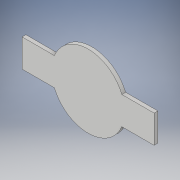
# Autodesk Inventor part: Emblem
Saved by Autodesk Inventor 2019.3 (Build 233278000, 278)
## iProperties
Created: 2020-09-20
Part Number: Emblem
Material: Generisch
Document SubType Name: Modeling
Designer: Nicolas Frick
Density: 1 g/cm^3
Appearance: Vorgabe
Author: Nicolas Frick
Autodesk Inventor part; units mm, degrees
ref_plane "YZ Plane" through (0, 0, 0) normal (1, 0, 0) x (0, 1, 0)
ref_plane "XZ Plane" through (0, 0, 0) normal (0, 1, 0) x (-1, 0, 0)
ref_plane "XY Plane" through (0, 0, 0) normal (0, 0, 1) x (1, 0, 0)
sketch "Skizze1" plane through (0, 0, 0) normal (0, 0, 1) x (1, 0, 0)
  line L0 (-50, 9) -> (-50, -9) construction
  line L1 (50, 9) -> (50, -9) construction
  line L2 (-50, -9) -> (-50, 9)
  line L3 (-50, 9) -> (-25.1982, 9)
  line L4 (25.1982, 9) -> (50, 9)
  line L5 (50, -9) -> (25.1982, -9)
  line L6 (-25.1982, -9) -> (-50, -9)
  line L7 (50, 9) -> (29.5255, 5.3146) construction
  arc A0 (25.1982, 9) -> (-25.1982, 9) centre (0, 0) ccw
  arc A1 (-25.1982, -9) -> (25.1982, -9) centre (0, 0) ccw
  line L8 (50, -12.5) -> (50, -9) construction
  line L9 (50, 9) -> (50, 12.5) construction
  line L10 (50, 9) -> (50, -9)
  point P0 (0, 0)
  dimension "d13" = 100
  dimension "d14" = 18
  constraints: 22 end point, 7 parallel, 4 point on circle, 2 centre point, 2 horizontal, 2 perpendicular, 1 coincident, 1 collinear
  measures "d13" distance of L0.end L1.end
  measures "d14" distance of L1.start L1.end
extrude "Extrusion1" add sketch "Skizze1" along normal blind 3
sketch "Skizze3" plane through (0, 0, 0) normal (0, 0, -1) x (-1, 0, 0)
  line L0 (50, -12.5) -> (50, 12.5) construction
  line L1 (50, 12.5) -> (27.2718, 12.5) construction
  arc A0 (27.2718, 12.5) -> (-27.2718, 12.5) centre (0, 0) ccw construction
  line L2 (-27.2718, 12.5) -> (-50, 12.5) construction
  line L3 (-50, 12.5) -> (-50, -12.5) construction
  line L4 (-50, -12.5) -> (-27.2718, -12.5) construction
  arc A1 (-27.2718, -12.5) -> (27.2718, -12.5) centre (0, 0) ccw construction
  line L5 (27.2718, -12.5) -> (50, -12.5) construction
  line L6 (50, 9) -> (50, -9) projected
  line L7 (50, -9) -> (25.1982, -9) projected
  arc A2 (-25.1982, -9) -> (25.1982, -9) centre (0, 0) ccw projected
  line L8 (-25.1982, -9) -> (-50, -9) projected
  line L9 (-50, -9) -> (-50, 9) projected
  line L10 (-50, 9) -> (-25.1982, 9) projected
  arc A3 (25.1982, 9) -> (-25.1982, 9) centre (0, 0) ccw projected
  line L11 (25.1982, 9) -> (50, 9) projected
  line L12 (-26.5702, 11) -> (-52, 11)
  line L13 (-52, 11) -> (-52, -11)
  line L14 (-52, -11) -> (-26.5702, -11)
  arc A4 (-26.5702, -11) -> (26.5702, -11) centre (0, 0) ccw
  line L15 (26.5702, -11) -> (52, -11)
  line L16 (52, -11) -> (52, 11)
  line L17 (52, 11) -> (26.5702, 11)
  arc A5 (26.5702, 11) -> (-26.5702, 11) centre (0, 0) ccw
  dimension "d15" = 2
  constraints: 12 end point, 4 point on circle, 2 centre point, 7 other
  measures "d15" radial gap between concentric circles of A3 A5
extrude "Extrusion3" add sketch "Skizze3" against normal up to surface (3 mm away)
